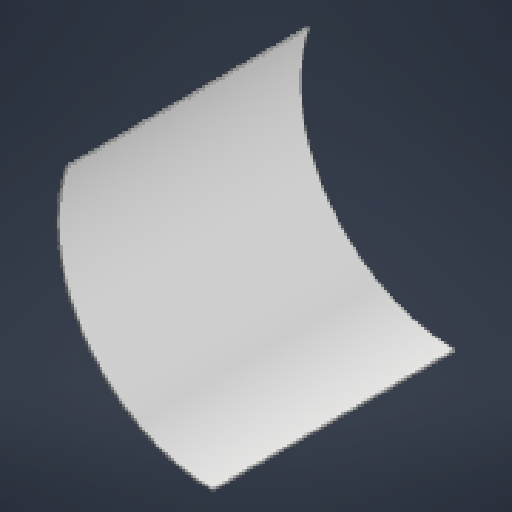
# Autodesk Inventor part: загиб 20-25
Saved by Autodesk Inventor 2025 (Build 290162000, 162)
## iProperties
Created: 2025-10-03
Part Number: загиб 20-25
Material: Типовые
Document SubType Name: Modeling
Designer: Phantom
Density: 1 g/cm^3
Appearance: По умолчанию
Author: Phantom
Autodesk Inventor part; units mm, degrees
ref_plane "YZ Plane" through (0, 0, 0) normal (1, 0, 0) x (0, 1, 0)
ref_plane "XZ Plane" through (0, 0, 0) normal (0, 1, 0) x (-1, 0, 0)
ref_plane "XY Plane" through (0, 0, 0) normal (0, 0, 1) x (1, 0, 0)
sketch "Эскиз1" plane through (0, 0, 0) normal (0, 0, 1) x (1, 0, 0)
  line L0 (9.8407, 227) -> (11.9652, 227)
  line L1 (220, 0) -> (230, 0) construction
  line L2 (0, 0) -> (170, 0)
  line L3 (170, 0) -> (170, 2)
  arc A0 (9.8407, 227) -> (170, 0) centre (170, 170) ccw
  arc A1 (11.9652, 227) -> (170, 2) centre (170, 170) ccw
  line L4 (170, 1) -> (170, 0)
  dimension "d12" = 340
  dimension "d13" = 2
  constraints: 10 end point, 4 point on circle, 2 centre point, 2 horizontal, 1 midpoint, 1 vertical
  measures "d12" diameter of A0
  measures "d13" radial gap between concentric circles of A0 A1
extrude "Выдавливание1" add sketch "Эскиз1" along normal blind 385
sketch "Эскиз2" plane through (0, 0, 0) normal (0, 0, -1) x (-1, 0, 0)
  line L0 (-11.9652, 227) -> (-9.8407, 227) projected
  arc A0 (-170, 2) -> (-11.9652, 227) centre (-170, 170) ccw projected
  line L1 (-170, 0) -> (-170, 2) projected
  arc A1 (-170, 0) -> (-9.8407, 227) centre (-170, 170) ccw projected
  point P0 (0, 0)
extrude "Выдавливание2" cut sketch "Эскиз2" against normal blind 121
chamfer "Фаска1" distance 2 angle 45 1 edges at (170, 2, 253)
chamfer "Фаска2" distance 2.8 angle 45 1 edges at (168.0001, 2.0119, 253)
